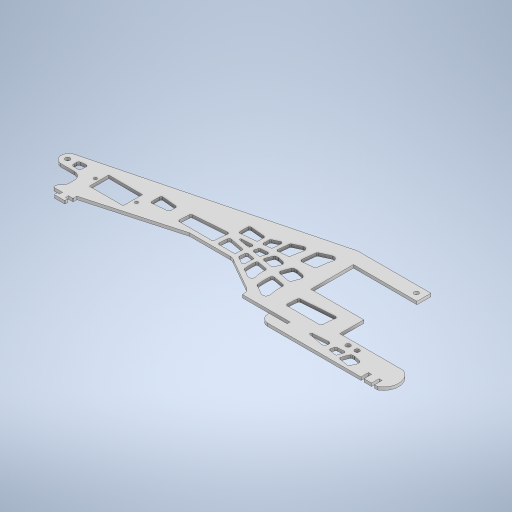
# Autodesk Inventor part: carbon_body
Saved by Autodesk Inventor 2024 (Build 280153000, 153)
## iProperties
Created: 2024-04-07
Part Number: carbon_body
Material: Generic
Document SubType Name: Modeling
Designer: nikop
Density: 1 g/cm^3
Appearance: Default
Author: nikop
Autodesk Inventor part; units mm, degrees
ref_plane "YZ Plane" through (0, 0, 0) normal (1, 0, 0) x (0, 1, 0)
ref_plane "XZ Plane" through (0, 0, 0) normal (0, 1, 0) x (-1, 0, 0)
ref_plane "XY Plane" through (0, 0, 0) normal (0, 0, 1) x (1, 0, 0)
sketch "Sketch1" plane through (0, 0, 0) normal (0, 1, 0) x (-1, 0, 0)
  line L0 (121.8515, 8.5991) -> (121.8515, 8.6002)
  line L1 (106.3006, 26.324) -> (106.3006, 25.1524)
  line L2 (105.8006, 26.824) -> (100.1932, 26.824)
  line L3 (96.1932, 28.8333) -> (94.9932, 28.8342)
  line L4 (101.3932, 28.8333) -> (100.1932, 28.8333)
  line L5 (94.6932, 29.1333) -> (94.6932, 30.5333)
  line L6 (101.6932, 29.1333) -> (101.6932, 30.5333)
  line L7 (96.1932, 28.8333) -> (94.9932, 28.8333)
  arc A0 (94.6932, 29.1333) -> (94.9932, 28.8333) centre (94.9932, 29.1333) ccw
  arc A1 (94.9932, 30.8333) -> (94.6932, 30.5333) centre (94.9932, 30.5333) ccw
  arc A2 (101.6932, 30.5333) -> (101.3932, 30.8333) centre (101.3932, 30.5333) ccw
  arc A3 (101.3932, 28.8333) -> (101.6932, 29.1333) centre (101.3932, 29.1333) ccw
  line L8 (117.6923, 10.824) -> (108.1923, 10.824)
  line L9 (106.3006, 26.324) -> (106.3006, 25.824)
  line L10 (105.7148, 23.7382) -> (104.6568, 22.6802)
  line L11 (103.1923, 15.824) -> (103.1923, 19.1447)
  arc A4 (104.6568, 22.6802) -> (103.1923, 19.1447) centre (108.1923, 19.1447) ccw
  arc A5 (103.1923, 15.824) -> (108.1923, 10.824) centre (108.1923, 15.824) ccw
  arc A6 (105.7148, 23.7382) -> (106.3006, 25.1524) centre (104.3006, 25.1524) ccw
  line L12 (93.1916, 26.324) -> (93.1916, 24.2428)
  line L13 (93.6916, 26.824) -> (96.1916, 26.824)
  arc A7 (93.6916, 26.824) -> (93.1916, 26.324) centre (93.6916, 26.324) ccw
  arc A8 (106.3006, 26.324) -> (105.8006, 26.824) centre (105.8006, 26.324) ccw
  arc A9 (-18.5458, 24.7704) -> (-16.1783, 20.6266) centre (-13.5469, 24.8781) ccw
  arc A10 (112.7487, 6.5727) -> (112.7487, 5.0753) centre (117.6923, 5.824) ccw
  line L14 (-9.2689, -7.3971) -> (-12.9832, -6.6002)
  arc A11 (-14.3597, -3.7646) -> (-13.082, -0.532) centre (-34.07, 5.8949) ccw
  arc A12 (5.0015, 8.5647) -> (7.5015, 7.8949) centre (7.5015, 12.8949) ccw
  arc A13 (-14.3597, -3.7646) -> (-12.9832, -6.6002) centre (-12.5637, -4.6447) ccw
  arc A14 (-9.9045, 13.7066) -> (-12.839, 11.4669) centre (-10.9045, 11.9746) ccw
  line L15 (111.3755, 8.2932) -> (108.1671, 8.5288)
  arc A15 (111.3755, 3.3547) -> (112.7487, 5.0753) centre (111.2656, 4.8507) ccw
  arc A16 (112.7487, 6.5727) -> (111.3755, 8.2932) centre (111.2656, 6.7973) ccw
  line L16 (111.3755, 3.3547) -> (108.1671, 3.1191)
  arc A17 (108.1671, 8.5288) -> (107.0938, 7.5315) centre (108.0938, 7.5315) ccw
  arc A18 (107.0938, 4.1165) -> (108.1671, 3.1191) centre (108.0938, 4.1165) ccw
  line L17 (111.3755, 3.3547) -> (108.1671, 3.1191)
  line L18 (-7.6969, -7.322) -> (-8.9859, -7.4166)
  line L19 (-7.6969, -7.322) -> (-8.9859, -7.4166)
  line L20 (1.6865, -6.6329) -> (-2.6626, -6.9523)
  line L21 (1.6865, -6.6329) -> (-2.6626, -6.9523)
  line L22 (1.6865, -6.6329) -> (-2.6626, -6.9523)
  line L23 (1.6865, -6.6329) -> (-2.6626, -6.9523)
  line L24 (1.6865, -6.6329) -> (-2.6626, -6.9523)
  line L25 (1.6865, -6.6329) -> (-2.6626, -6.9523)
  line L26 (1.6865, -6.6329) -> (-2.6626, -6.9523)
  line L27 (1.6865, -6.6329) -> (-2.6626, -6.9523)
  line L28 (1.6865, -6.6329) -> (-2.6626, -6.9523)
  line L29 (1.6865, -6.6329) -> (-2.6626, -6.9523)
  line L30 (-7.6969, -7.322) -> (-8.9859, -7.4166)
  line L31 (-7.6969, -7.322) -> (-8.9859, -7.4166)
  line L32 (-7.6969, -7.322) -> (-8.9859, -7.4166)
  line L33 (-7.6969, -7.322) -> (-8.9859, -7.4166)
  line L34 (-7.6969, -7.322) -> (-8.9859, -7.4166)
  line L35 (-7.6969, -7.322) -> (-8.9859, -7.4166)
  line L36 (-7.6969, -7.322) -> (-8.9859, -7.4166)
  line L37 (-7.6969, -7.322) -> (-8.9859, -7.4166)
  line L38 (17.6085, -5.4637) -> (17.5429, -5.4685)
  line L39 (17.6085, -5.4637) -> (17.5429, -5.4685)
  line L40 (17.6085, -5.4637) -> (17.5429, -5.4685)
  line L41 (17.6085, -5.4637) -> (17.5429, -5.4685)
  line L42 (17.6085, -5.4637) -> (17.5429, -5.4685)
  line L43 (17.6085, -5.4637) -> (17.5429, -5.4685)
  line L44 (17.6085, -5.4637) -> (17.5429, -5.4685)
  line L45 (17.6085, -5.4637) -> (17.5429, -5.4685)
  line L46 (17.6085, -5.4637) -> (17.5429, -5.4685)
  line L47 (13.8135, -5.7424) -> (7.0175, -6.2415)
  line L48 (44.0726, -3.5204) -> (26.4909, -4.8115)
  line L49 (44.0726, -3.5204) -> (26.4909, -4.8115)
  line L50 (44.0726, -3.5204) -> (26.4909, -4.8115)
  line L51 (44.0726, -3.5204) -> (26.4909, -4.8115)
  line L52 (44.0726, -3.5204) -> (26.4909, -4.8115)
  line L53 (44.0726, -3.5204) -> (26.4909, -4.8115)
  line L54 (44.0726, -3.5204) -> (26.4909, -4.8115)
  line L55 (44.0726, -3.5204) -> (26.4909, -4.8115)
  line L56 (44.0726, -3.5204) -> (26.4909, -4.8115)
  line L57 (44.0726, -3.5204) -> (22.1244, -5.1321)
  line L58 (7.3285, -3.508) -> (13.8703, -4.7526)
  line L59 (-1.5324, -1.8222) -> (2.4069, -2.5717)
  line L60 (-11.9389, 0.1576) -> (-5.9674, -0.9785)
  line L61 (7.8892, -0.5609) -> (17.2299, -2.3379)
  line L62 (-0.9717, 1.1249) -> (2.9676, 0.3755)
  line L63 (-11.3782, 3.1047) -> (-5.4067, 1.9687)
  arc A19 (-12.1882, 4.1659) -> (-12.839, 11.4669) centre (-34.07, 5.8949) ccw
  arc A20 (-12.1882, 4.1659) -> (-11.3782, 3.1047) centre (-11.1913, 4.0871) ccw
  arc A21 (-11.9389, 0.1576) -> (-13.082, -0.532) centre (-12.1258, -0.8248) ccw
  arc A22 (-5.1917, -2.2318) -> (-5.9674, -0.9785) centre (-6.1543, -1.9609) ccw
  arc A23 (-9.2689, -7.3971) -> (-8.9859, -7.4166) centre (-9.0591, -6.4193) ccw
  arc A24 (-7.6969, -7.322) -> (-6.8632, -6.746) centre (-7.7701, -6.3247) ccw
  arc A25 (-3.6712, -5.6012) -> (-2.6626, -6.9523) centre (-2.7358, -5.955) ccw
  arc A26 (-1.5324, -1.8222) -> (-2.685, -2.5449) centre (-1.7193, -2.8046) ccw
  arc A27 (3.1878, -3.806) -> (2.4069, -2.5717) centre (2.22, -3.5541) ccw
  arc A28 (1.6865, -6.6329) -> (2.5649, -5.9431) centre (1.6133, -5.6356) ccw
  arc A29 (5.9793, -4.982) -> (7.0175, -6.2415) centre (6.9443, -5.2441) ccw
  arc A30 (7.3285, -3.508) -> (6.1719, -4.246) centre (7.1416, -4.4904) ccw
  arc A31 (-1.7784, 2.2203) -> (-0.9717, 1.1249) centre (-0.7848, 2.1073) ccw
  arc A32 (2.9676, 0.3755) -> (4.1472, 1.2368) centre (3.1545, 1.3578) ccw
  arc A33 (4.4154, 4.8339) -> (3.9158, 5.7275) centre (3.4158, 4.8615) ccw
  arc A34 (-0.0945, 8.0428) -> (-1.5938, 7.1385) centre (-0.5945, 7.1768) ccw
  arc A35 (-4.3608, 10.0619) -> (-4.8511, 10.789) centre (-5.3511, 9.923) ccw
  arc A36 (8.3829, 4.8949) -> (7.384, 3.9419) centre (8.3829, 3.8949) ccw
  arc A37 (18.8784, 3.8529) -> (17.8793, 4.8949) centre (17.8793, 3.8949) ccw
  arc A38 (17.2299, -2.3379) -> (18.4079, -1.4888) centre (17.4168, -1.3555) ccw
  arc A39 (-5.4067, 1.9687) -> (-4.225, 2.8495) centre (-5.2198, 2.951) ccw
  arc A40 (13.8135, -5.7424) -> (13.8703, -4.7526) centre (13.7769, -5.2438) ccw
  line L64 (13.8135, -5.7424) -> (7.0175, -6.2415)
  line L65 (13.8135, -5.7424) -> (7.0175, -6.2415)
  line L66 (13.8135, -5.7424) -> (7.0175, -6.2415)
  line L67 (13.8135, -5.7424) -> (7.0175, -6.2415)
  line L68 (13.8135, -5.7424) -> (7.0175, -6.2415)
  line L69 (13.8135, -5.7424) -> (7.0175, -6.2415)
  line L70 (13.8135, -5.7424) -> (7.0175, -6.2415)
  line L71 (13.8135, -5.7424) -> (7.0175, -6.2415)
  line L72 (13.8135, -5.7424) -> (7.0175, -6.2415)
  line L73 (24.4215, 4.8949) -> (22.8833, 4.8949)
  line L74 (17.8793, 4.8949) -> (8.3829, 4.8949)
  arc A41 (7.0844, 0.5503) -> (7.8892, -0.5609) centre (8.0761, 0.4215) ccw
  line L75 (44.4058, 4.8949) -> (24.4215, 4.8949)
  arc A42 (22.8833, 4.8949) -> (21.8841, 3.9335) centre (22.8833, 3.8949) ccw
  arc A43 (21.0652, -3.9677) -> (22.1244, -5.1321) centre (22.0511, -4.1348) ccw
  arc A44 (44.0726, -3.5204) -> (44.9942, -2.6251) centre (43.9994, -2.5231) ccw
  arc A45 (45.4055, 3.8706) -> (44.4058, 4.8949) centre (44.4058, 3.8949) ccw
  line L76 (3.9158, 5.7275) -> (-0.0945, 8.0428)
  line L77 (-4.8511, 10.789) -> (-9.9045, 13.7066)
  line L78 (107.0938, 7.5315) -> (107.0938, 4.1165)
  arc A46 (-6.8632, -6.746) -> (-5.1917, -2.2318) centre (-34.07, 5.8949) ccw
  arc A47 (-4.225, 2.8495) -> (-4.3608, 10.0619) centre (-34.07, 5.8949) ccw
  arc A48 (-3.6712, -5.6012) -> (-2.685, -2.5449) centre (-34.07, 5.8949) ccw
  arc A49 (-1.7784, 2.2203) -> (-1.5938, 7.1385) centre (-34.07, 5.8949) ccw
  arc A50 (18.4079, -1.4888) -> (18.8784, 3.8529) centre (-39.57, 6.3096) ccw
  arc A51 (21.0652, -3.9677) -> (21.8841, 3.9335) centre (-39.57, 6.3096) ccw
  arc A52 (21.8975, 8.3096) -> (21.8958, 8.3596) centre (-39.57, 6.3096) ccw
  arc A53 (44.9942, -2.6251) -> (45.4055, 3.8706) centre (-38.07, 5.8949) ccw
  arc A54 (48.4068, 7.9178) -> (48.406, 7.9531) centre (-38.0701, 5.9178) ccw
  arc A55 (2.5649, -5.9431) -> (3.1878, -3.806) centre (-34.07, 5.8949) ccw
  arc A56 (4.1472, 1.2368) -> (4.4154, 4.8339) centre (-34.07, 5.8949) ccw
  arc A57 (4.4272, 5.4322) -> (4.4273, 5.44) centre (-34.07, 5.8949) ccw
  arc A58 (5.9793, -4.982) -> (6.1719, -4.246) centre (-34.07, 5.8949) ccw
  arc A59 (7.0844, 0.5503) -> (7.384, 3.9419) centre (-34.07, 5.8949) ccw
  line L79 (94.9932, 30.8333) -> (101.3932, 30.8333)
  line L80 (-18.5458, 24.8943) -> (-18.5458, 24.7704)
  line L81 (94.7702, 1.4979) -> (72.2704, 1.6071)
  line L82 (94.7702, 1.4979) -> (94.7702, 14.4023)
  line L83 (94.7702, 14.4023) -> (72.2702, 14.4018)
  line L84 (72.2702, 14.4018) -> (72.2704, 1.6071)
  circle A60 centre (117.6828, 5.8842) radius 1.55
  line L85 (-73.5399, 16.0427) -> (-114.5899, 16.0427)
  line L86 (7.5015, 7.8949) -> (34.5015, 7.8949)
  line L87 (-50.2842, 25.8335) -> (-18.5458, 25.8335)
  line L88 (-18.5458, 25.8335) -> (-18.5458, 24.7704)
  line L89 (-26.2577, 6.5958) -> (-19.0919, 5.2325)
  arc A61 (-17.8368, 14.9444) -> (-18.4252, 15.817) centre (-19.0252, 14.7778) ccw
  arc A62 (-19.0919, 5.2325) -> (-17.6738, 6.2896) centre (-18.8676, 6.4114) ccw
  arc A63 (-17.6738, 6.2896) -> (-17.8368, 14.9444) centre (-53.4879, 9.944) ccw
  line L90 (-18.4252, 15.817) -> (-24.4893, 19.3181)
  arc A64 (-27.2297, 7.8692) -> (-26.2577, 6.5958) centre (-26.0334, 7.7747) ccw
  arc A65 (-27.2297, 7.8692) -> (-28.0107, 16.6304) centre (-53.4879, 9.944) ccw
  arc A66 (-24.4893, 19.3181) -> (-28.0107, 16.6304) centre (-25.6893, 17.2396) ccw
  line L91 (-20.8522, -6.3271) -> (-22.399, -6.4406)
  line L92 (-20.8522, -6.3271) -> (-22.399, -6.4406)
  line L93 (-20.8522, -6.3271) -> (-22.399, -6.4406)
  line L94 (-20.8522, -6.3271) -> (-22.399, -6.4406)
  line L95 (-25.9426, 2.6484) -> (-18.7768, 1.2851)
  line L96 (-20.8522, -6.3271) -> (-22.399, -6.4406)
  line L97 (-22.7386, -6.4172) -> (-27.1958, -5.461)
  arc A67 (-28.8476, -2.0582) -> (-27.1958, -5.461) centre (-26.6924, -3.1144) ccw
  arc A68 (-28.8476, -2.0582) -> (-27.3143, 1.8209) centre (-52.5, 9.5332) ccw
  line L98 (-20.8522, -6.3271) -> (-22.399, -6.4406)
  line L99 (-20.8522, -6.3271) -> (-22.399, -6.4406)
  line L100 (-20.8522, -6.3271) -> (-22.399, -6.4406)
  line L101 (-20.8522, -6.3271) -> (-22.399, -6.4406)
  line L102 (-20.8522, -6.3271) -> (-22.399, -6.4406)
  arc A69 (-19.8518, -5.6359) -> (-17.846, -0.2188) centre (-52.5, 9.5332) ccw
  arc A70 (-20.8522, -6.3271) -> (-19.8518, -5.6359) centre (-20.9401, -5.1303) ccw
  arc A71 (-17.846, -0.2188) -> (-18.7768, 1.2851) centre (-19.0011, 0.1063) ccw
  arc A72 (-22.7386, -6.4172) -> (-22.399, -6.4406) centre (-22.4869, -5.2439) ccw
  arc A73 (-25.9426, 2.6484) -> (-27.3143, 1.8209) centre (-26.1669, 1.4695) ccw
  line L103 (-73.5399, 16.0427) -> (-81.0399, 16.0427)
  line L104 (-73.5399, 16.0427) -> (-81.0399, 16.0427)
  arc A74 (-38.2842, 28.8335) -> (-43.3456, 33.8949) centre (-43.2838, 28.8953) ccw
  line L105 (-74.5399, 33.8949) -> (-43.3456, 33.8949)
  line L106 (-100.5399, 33.8949) -> (-98.5399, 33.8949)
  circle A75 centre (-89.0399, 20.0427) radius 1.525
  circle A76 centre (-83.0399, 20.0427) radius 1.525
  line L107 (-100.5399, 33.8949) -> (-98.5399, 33.8949) construction
  line L108 (-100.5399, 33.8949) -> (-104.5399, 33.8949)
  line L109 (-107.5399, 28.8949) -> (-107.5399, 33.8949)
  line L110 (-107.5399, 33.8949) -> (-112.5399, 33.8949)
  line L111 (-112.5399, 33.8949) -> (-112.5399, 28.8949)
  line L112 (-114.5399, 33.8949) -> (-116.5399, 33.8949)
  line L113 (-114.5899, 16.0427) -> (-116.0399, 16.0427)
  arc A77 (-116.5399, 33.8949) -> (-116.0399, 16.0427) centre (-111.7902, 25.0948) ccw
  circle A78 centre (97.2702, 7.9501) radius 1.05
  circle A79 centre (69.7703, 8.0044) radius 1.05
  line L114 (-80.5399, -37.5874) -> (-31.7565, -37.5874)
  line L115 (-80.5399, -37.5874) -> (-80.5399, -28.3154)
  line L116 (-80.5399, -28.3154) -> (-38.2842, -28.3154)
  circle A80 centre (-75.5399, -32.9514) radius 1.525
  line L117 (-73.5399, 16.0427) -> (-73.5399, 1.0427)
  line L118 (-73.5399, 1.0427) -> (-73.5399, 0.0427)
  line L119 (-73.5399, 1.0427) -> (-72.5399, 1.0427) construction
  line L120 (-73.5399, 0.0427) -> (-38.2842, 0.0427)
  line L121 (-38.2842, 0.0427) -> (-38.2842, -28.3154)
  line L122 (-26.7273, -13.5092) -> (-19.4671, -12.8044)
  arc A81 (-26.7273, -13.5092) -> (-27.8113, -14.6888) centre (-26.6114, -14.7036) ccw
  arc A82 (-29.3871, -23.3424) -> (-26.1251, -26.3397) centre (-27.1308, -24.1606) ccw
  line L123 (-19.7674, -23.4056) -> (-26.1251, -26.3397)
  arc A83 (-19.7674, -23.4056) -> (-19.102, -22.5902) centre (-20.2702, -22.316) ccw
  arc A84 (-18.1512, -13.9862) -> (-19.4671, -12.8044) centre (-19.3512, -13.9987) ccw
  arc A85 (-4.4449, -11.7855) -> (-5.5415, -10.8007) centre (-5.4449, -11.796) ccw
  line L124 (-11.5917, -11.3881) -> (-5.5415, -10.8007)
  arc A86 (-11.5917, -11.3881) -> (-12.495, -12.371) centre (-11.4951, -12.3834) ccw
  arc A87 (-13.8081, -19.5824) -> (-11.0898, -22.0801) centre (-11.9279, -20.2642) ccw
  line L125 (-5.7917, -19.635) -> (-11.0898, -22.0801)
  arc A88 (-5.7917, -19.635) -> (-5.2372, -18.9555) centre (-6.2107, -18.727) ccw
  line L126 (-1.0481, -10.3644) -> (2.9431, -9.9769)
  arc A89 (-1.0481, -10.3644) -> (-1.9512, -11.3818) centre (-0.9515, -11.3597) ccw
  arc A90 (-2.2154, -16.2964) -> (-0.8047, -17.3335) centre (-1.2238, -16.4255) ccw
  arc A91 (3.3998, -15.393) -> (3.9787, -14.5487) centre (2.9808, -14.4851) ccw
  arc A92 (4.0393, -10.9422) -> (2.9431, -9.9769) centre (3.0398, -10.9722) ccw
  arc A93 (7.0163, -13.9308) -> (7.0269, -10.526) centre (-34.4433, -12.0996) ccw
  arc A94 (7.9295, -9.4928) -> (7.0269, -10.526) centre (8.0261, -10.4881) ccw
  line L127 (7.9295, -9.4928) -> (17.3933, -8.574)
  arc A95 (7.0163, -13.9308) -> (7.9242, -14.9708) centre (8.0153, -13.975) ccw
  line L128 (17.3811, -15.8358) -> (7.9242, -14.9708)
  arc A96 (17.3811, -15.8358) -> (18.471, -14.8892) centre (17.4722, -14.84) ccw
  arc A97 (18.471, -14.8892) -> (18.489, -9.5268) centre (-39.9582, -12.0116) ccw
  arc A98 (18.489, -9.5268) -> (17.3933, -8.574) centre (17.4899, -9.5693) ccw
  line L129 (3.3998, -15.393) -> (-0.8047, -17.3335)
  line L130 (-28.5902, -20.5804) -> (-29.3871, -23.3424)
  line L131 (-50.2842, 25.8335) -> (-50.2842, 27.8335)
  line L132 (-50.2842, 27.8335) -> (-38.2842, 27.8335)
  line L133 (-38.2842, 27.8335) -> (-38.2842, 28.8335)
  line L134 (-112.5399, 28.8949) -> (-114.5399, 28.8949)
  line L135 (-114.5399, 28.8949) -> (-114.5399, 33.8949)
  line L136 (-107.5399, 28.8949) -> (-105.5399, 28.8949)
  line L137 (-105.5399, 28.8949) -> (-105.5399, 33.8949)
  line L138 (-105.5399, 33.8949) -> (-104.5399, 33.8949)
  line L139 (-40.332, 9.1498) -> (-57.9138, 7.8587)
  line L140 (-40.332, 9.1498) -> (-57.9138, 7.8587)
  line L141 (-40.332, 9.1498) -> (-57.9138, 7.8587)
  line L142 (-40.332, 9.1498) -> (-57.9138, 7.8587)
  line L143 (-40.332, 9.1498) -> (-62.2803, 7.5381)
  line L144 (-40.332, 9.1498) -> (-57.9138, 7.8587)
  line L145 (-40.332, 9.1498) -> (-57.9138, 7.8587)
  line L146 (-40.332, 9.1498) -> (-57.9138, 7.8587)
  line L147 (-40.332, 9.1498) -> (-57.9138, 7.8587)
  line L148 (-40.332, 9.1498) -> (-57.9138, 7.8587)
  arc A99 (-39.4105, 10.0451) -> (-38.9992, 16.5408) centre (-122.4747, 18.5651) ccw
  arc A100 (-40.332, 9.1498) -> (-39.4105, 10.0451) centre (-40.4053, 10.1471) ccw
  arc A101 (-38.9992, 16.5408) -> (-39.9989, 17.5651) centre (-39.9989, 16.5651) ccw
  line L149 (-39.9989, 17.5651) -> (-59.9832, 17.5651)
  arc A102 (-63.3395, 8.7025) -> (-62.2803, 7.5381) centre (-62.3535, 8.5354) ccw
  line L150 (-59.9832, 17.5651) -> (-61.5213, 17.5651)
  arc A103 (-63.3395, 8.7025) -> (-62.5206, 16.6037) centre (-123.9747, 18.9798) ccw
  arc A104 (-61.5213, 17.5651) -> (-62.5206, 16.6037) centre (-61.5213, 16.5651) ccw
  arc A105 (-85.986, 25.9679) -> (-84.9998, 29.0242) centre (-116.3848, 37.464) ccw
  arc A106 (-89.178, 24.8231) -> (-87.5065, 29.3374) centre (-116.3848, 37.464) ccw
  arc A107 (-79.7499, 25.6261) -> (-79.127, 27.7631) centre (-116.3848, 37.464) ccw
  line L151 (-90.0117, 24.2472) -> (-91.3007, 24.1525)
  line L152 (-90.0117, 24.2472) -> (-91.3007, 24.1525)
  line L153 (-90.0117, 24.2472) -> (-91.3007, 24.1525)
  line L154 (-90.0117, 24.2472) -> (-91.3007, 24.1525)
  line L155 (-90.0117, 24.2472) -> (-91.3007, 24.1525)
  line L156 (-90.0117, 24.2472) -> (-91.3007, 24.1525)
  line L157 (-90.0117, 24.2472) -> (-91.3007, 24.1525)
  line L158 (-90.0117, 24.2472) -> (-91.3007, 24.1525)
  line L159 (-90.0117, 24.2472) -> (-91.3007, 24.1525)
  line L160 (-80.6283, 24.9362) -> (-84.9774, 24.6169)
  line L161 (-80.6283, 24.9362) -> (-84.9774, 24.6169)
  line L162 (-80.6283, 24.9362) -> (-84.9774, 24.6169)
  line L163 (-80.6283, 24.9362) -> (-84.9774, 24.6169)
  line L164 (-80.6283, 24.9362) -> (-84.9774, 24.6169)
  line L165 (-80.6283, 24.9362) -> (-84.9774, 24.6169)
  line L166 (-80.6283, 24.9362) -> (-84.9774, 24.6169)
  line L167 (-80.6283, 24.9362) -> (-84.9774, 24.6169)
  line L168 (-80.6283, 24.9362) -> (-84.9774, 24.6169)
  line L169 (-83.8472, 29.7469) -> (-79.9079, 28.9975)
  arc A108 (-80.6283, 24.9362) -> (-79.7499, 25.6261) centre (-80.7015, 25.9335) ccw
  line L170 (-80.6283, 24.9362) -> (-84.9774, 24.6169)
  line L171 (-91.5837, 24.1721) -> (-95.298, 24.9689)
  arc A109 (-96.6745, 27.8045) -> (-95.3968, 31.0371) centre (-116.3848, 37.464) ccw
  arc A110 (-96.6745, 27.8045) -> (-95.298, 24.9689) centre (-94.8786, 26.9244) ccw
  arc A111 (-91.5837, 24.1721) -> (-91.3007, 24.1525) centre (-91.3739, 25.1498) ccw
  line L172 (-90.0117, 24.2472) -> (-91.3007, 24.1525)
  arc A112 (-79.127, 27.7631) -> (-79.9079, 28.9975) centre (-80.0948, 28.0151) ccw
  line L173 (-94.2537, 31.7267) -> (-88.2822, 30.5907)
  arc A113 (-94.2537, 31.7267) -> (-95.3968, 31.0371) centre (-94.4406, 30.7443) ccw
  arc A114 (-87.5065, 29.3374) -> (-88.2822, 30.5907) centre (-88.4691, 29.6083) ccw
  arc A115 (-83.8472, 29.7469) -> (-84.9998, 29.0242) centre (-84.0341, 28.7645) ccw
  arc A116 (-85.986, 25.9679) -> (-84.9774, 24.6169) centre (-85.0506, 25.6142) ccw
  arc A117 (-90.0117, 24.2472) -> (-89.178, 24.8231) centre (-90.0849, 25.2445) ccw
  line L174 (-73.9133, 28.3344) -> (-64.1005, 26.4675)
  arc A118 (-73.9133, 28.3344) -> (-75.6481, 27.2273) centre (-74.1936, 26.8608) ccw
  arc A119 (-75.9406, 26.11) -> (-74.3797, 24.2342) centre (-74.4895, 25.7301) ccw
  line L175 (-64.1858, 24.9827) -> (-74.3797, 24.2342)
  arc A120 (-64.1858, 24.9827) -> (-64.1005, 26.4675) centre (-64.2407, 25.7307) ccw
  line L176 (-75.6481, 27.2273) -> (-75.9406, 26.11)
  arc A121 (64.0621, -3.8679) -> (65.152, -2.9213) centre (64.1532, -2.8721) ccw
  line L177 (64.0621, -3.8679) -> (54.6053, -3.0029)
  arc A122 (65.152, -2.9213) -> (65.17, 2.4411) centre (6.7228, -0.0437) ccw
  arc A123 (65.17, 2.4411) -> (64.0743, 3.3939) centre (64.1709, 2.3986) ccw
  line L178 (54.6105, 2.4751) -> (64.0743, 3.3939)
  arc A124 (53.6973, -1.9629) -> (53.7079, 1.4419) centre (12.2377, -0.1317) ccw
  arc A125 (54.6105, 2.4751) -> (53.7079, 1.4419) centre (54.7072, 1.4798) ccw
  arc A126 (53.6973, -1.9629) -> (54.6053, -3.0029) centre (54.6963, -2.0071) ccw
  line L179 (117.6923, 0.824) -> (-31.7565, -37.5874)
  line L180 (34.5015, 7.8949) -> (93.1916, 24.2428)
  line L181 (-16.1783, 20.6266) -> (5.0015, 8.5647)
  line L182 (-98.5399, 33.8949) -> (-74.5399, 33.8949)
  arc A127 (117.6923, 0.824) -> (117.6923, 10.824) centre (116.9653, 5.824) ccw
  line L183 (100.1932, 26.824) -> (100.1932, 28.8333)
  line L184 (96.1916, 26.824) -> (96.1932, 28.8333)
  line L185 (-2.2154, -16.1914) -> (-2.2154, -16.2964)
  line L186 (-2.2154, -16.1914) -> (-1.9512, -11.3818)
  line L187 (-12.495, -12.371) -> (-13.8081, -19.5824)
  line L188 (-4.4449, -11.7855) -> (-5.2372, -18.9555)
  line L189 (-28.5902, -20.5804) -> (-27.8113, -14.6888)
  line L190 (-18.1512, -13.9862) -> (-19.102, -22.5902)
  line L191 (4.0393, -10.9422) -> (3.9787, -14.5487)
  point P0 (0, 0)
  point P1 (93.1916, 26.324)
  point P2 (104.6568, 22.6802)
  point P3 (94.6932, 30.5333)
  point P4 (94.6932, 29.1333)
  point P5 (94.9929, 28.8333)
  point P6 (-85.986, 25.9679)
  point P7 (-84.9998, 29.0242)
  point P8 (-83.8472, 29.7469)
  point P9 (-79.127, 27.7631)
  point P10 (-79.7499, 25.6261)
  point P11 (-95.298, 24.9689)
  point P12 (-95.3968, 31.0371)
  point P13 (-94.2537, 31.7267)
  point P14 (-88.2822, 30.5907)
  point P15 (-87.5065, 29.3374)
  point P16 (-89.178, 24.8231)
  point P17 (-22.7386, -6.4172)
  point P18 (-28.8476, -2.0582)
  point P19 (-27.3143, 1.8209)
  point P20 (-18.7768, 1.2851)
  point P21 (-17.846, -0.2188)
  point P22 (-19.8518, -5.6359)
  point P23 (-9.2689, -7.3971)
  point P24 (-12.9832, -6.6002)
  point P25 (-14.3597, -3.7646)
  point P26 (-13.082, -0.532)
  point P27 (-11.9389, 0.1576)
  point P28 (-5.9674, -0.9785)
  point P29 (-5.1917, -2.2318)
  point P30 (-6.8632, -6.746)
  point P31 (-3.6712, -5.6012)
  point P32 (-2.685, -2.5449)
  point P33 (3.1878, -3.806)
  point P34 (2.5649, -5.9431)
  point P35 (21.0652, -3.9677)
  point P36 (21.8841, 3.9335)
  point P37 (45.4055, 3.8706)
  point P38 (44.9942, -2.6251)
  point P39 (107.0938, 4.1165)
  point P40 (107.0938, 7.5315)
  point P41 (112.7487, 6.5727)
  point P42 (112.7487, 5.0753)
  point P43 (-63.3395, 8.7025)
  point P44 (-62.5206, 16.6037)
  point P45 (-38.9992, 16.5408)
  point P46 (-39.4105, 10.0451)
  point P47 (-19.7674, -23.4056)
  point P48 (53.7079, 1.4419)
  point P49 (54.6105, 2.4751)
  point P50 (65.17, 2.4411)
  point P51 (65.152, -2.9213)
  point P52 (-28.0107, 16.6304)
  point P53 (-18.4252, 15.817)
  point P54 (-17.8368, 14.9444)
  point P55 (-17.6738, 6.2896)
  point P56 (-26.2577, 6.5958)
  point P57 (7.0844, 0.5503)
  point P58 (7.384, 3.9419)
  point P59 (17.8793, 4.8949)
  point P60 (18.8784, 3.8529)
  point P61 (18.4079, -1.4888)
  point P62 (-1.7784, 2.2203)
  point P63 (-1.5938, 7.1385)
  point P64 (-0.0945, 8.0428)
  point P65 (3.9158, 5.7275)
  point P66 (4.4154, 4.8339)
  point P67 (4.1472, 1.2368)
  point P68 (-12.1882, 4.1659)
  point P69 (-12.839, 11.4669)
  point P70 (-4.8511, 10.789)
  point P71 (-4.3608, 10.0619)
  point P72 (-4.225, 2.8495)
  point P73 (-5.4067, 1.9687)
  point P74 (-11.3782, 3.1047)
  point P75 (17.3811, -15.8358)
  point P76 (7.0163, -13.9308)
  point P77 (7.0269, -10.526)
  point P78 (17.3933, -8.574)
  point P79 (18.489, -9.5268)
  point P80 (18.471, -14.8892)
  point P81 (-1.0481, -10.3644)
  point P82 (3.3998, -15.393)
  point P83 (-11.0898, -22.0801)
  point P84 (-11.5917, -11.3881)
  point P85 (-5.5415, -10.8007)
  point P86 (5.9793, -4.982)
  point P87 (6.1719, -4.246)
  dimension "d0" = 22.5
  dimension "d1" = 22.5
  dimension "d2" = 3.1
  dimension "d3" = 24
  dimension "d4" = 27
  dimension "d5" = 7.5
  dimension "d6" = 5
  dimension "d7" = 3.05
  dimension "d8" = 3.05
  dimension "d9" = 4
  dimension "d11" = 5
  dimension "d12" = 5
  dimension "d13" = 2
  dimension "d14" = 10
  dimension "d15" = 2.1
  dimension "d16" = 2.1
  dimension "d17" = 9.272
  dimension "d18" = 3.05
  dimension "d19" = 1
  dimension "d20" = 90
  dimension "d23" = 2
  dimension "d24" = 2
  dimension "d25" = 2
  constraints: 384 end point, 245 point on circle, 128 centre point, 10 horizontal, 9 perpendicular, 8 vertical, 5 point on line, 2 collinear, 1 tangent
  measures "d0" distance of L81.start L84.end
  measures "d1" distance of L82.end L84.start
  measures "d2" diameter of A60
  measures "d3" distance of L105.start L106.end
  measures "d4" distance of L86.start L86.end
  measures "d5" distance of L85.start L103.end
  measures "d6" radius of A74
  measures "d7" diameter of A75
  measures "d8" diameter of A76
  measures "d9" distance of L106.start L138.end
  measures "d11" distance of L110.start L110.end
  measures "d12" distance of L110.end L111.end
  measures "d13" distance of L135.end L112.end
  measures "d14" radius of A77
  measures "d15" diameter of A78
  measures "d16" diameter of A79
  measures "d17" distance of L114.start L116.start
  measures "d18" diameter of A80
  measures "d19" distance of L117.end L118.end
  measures "d20" angle of L118 L119
  measures "d23" distance of L87.start L131.end
  measures "d24" distance of L111.end L135.start
  measures "d25" distance of L109.start L136.end
extrude "Extrusion1" add sketch "Sketch1" along normal blind 2
body "Solid1"
